Autodesk Inventor part; units mm, degrees
(part 2 of 2)
  line L970 (21.6726, 19.3199) -> (21.796, 19.3518)
  line L971 (21.796, 19.3518) -> (21.9215, 19.3807)
  line L972 (21.9215, 19.3807) -> (22.0489, 19.4065)
  line L973 (22.0489, 19.4065) -> (22.1782, 19.4293)
  line L974 (22.1782, 19.4293) -> (22.4868, 18.9817)
  line L975 (22.4868, 18.9817) -> (22.4196, 18.8689)
  line L976 (22.4196, 18.8689) -> (22.3502, 18.759)
  line L977 (22.3502, 18.759) -> (22.2787, 18.6519)
  line L978 (22.2787, 18.6519) -> (22.2049, 18.5479)
  line L979 (22.2049, 18.5479) -> (22.129, 18.4471)
  line L980 (22.129, 18.4471) -> (22.0506, 18.3498)
  line L981 (22.0506, 18.3498) -> (21.9698, 18.2563)
  line L982 (21.9698, 18.2563) -> (21.8864, 18.1668)
  line L983 (21.8864, 18.1668) -> (21.8436, 18.1237)
  line L984 (21.8436, 18.1237) -> (21.8, 18.0819)
  line L985 (21.8, 18.0819) -> (21.7779, 18.0615)
  line L986 (21.7779, 18.0615) -> (21.7556, 18.0414)
  line L987 (21.7556, 18.0414) -> (21.733, 18.0218)
  line L988 (21.733, 18.0218) -> (21.7101, 18.0026)
  line L989 (21.7101, 18.0026) -> (22.0351, 17.4306)
  line L990 (22.0351, 17.4306) -> (22.0632, 17.4404)
  line L991 (22.0632, 17.4404) -> (22.0917, 17.4497)
  line L992 (22.0917, 17.4497) -> (22.1203, 17.4586)
  line L993 (22.1203, 17.4586) -> (22.1492, 17.4672)
  line L994 (22.1492, 17.4672) -> (22.2074, 17.4832)
  line L995 (22.2074, 17.4832) -> (22.2663, 17.4979)
  line L996 (22.2663, 17.4979) -> (22.3859, 17.5237)
  line L997 (22.3859, 17.5237) -> (22.5077, 17.5452)
  line L998 (22.5077, 17.5452) -> (22.6314, 17.5626)
  line L999 (22.6314, 17.5626) -> (22.7569, 17.5764)
  line L1000 (22.7569, 17.5764) -> (22.884, 17.5865)
  line L1001 (22.884, 17.5865) -> (23.0125, 17.5931)
  line L1002 (23.0125, 17.5931) -> (23.1425, 17.5964)
  line L1003 (23.1425, 17.5964) -> (23.2738, 17.5964)
  line L1004 (23.2738, 17.5964) -> (23.5001, 17.102)
  line L1005 (23.5001, 17.102) -> (23.4143, 17.0026)
  line L1006 (23.4143, 17.0026) -> (23.3269, 16.9063)
  line L1007 (23.3269, 16.9063) -> (23.2379, 16.8134)
  line L1008 (23.2379, 16.8134) -> (23.1472, 16.7238)
  line L1009 (23.1472, 16.7238) -> (23.0548, 16.6378)
  line L1010 (23.0548, 16.6378) -> (22.9608, 16.5555)
  line L1011 (22.9608, 16.5555) -> (22.8649, 16.4774)
  line L1012 (22.8649, 16.4774) -> (22.7672, 16.4037)
  line L1013 (22.7672, 16.4037) -> (22.7176, 16.3687)
  line L1014 (22.7176, 16.3687) -> (22.6674, 16.3351)
  line L1015 (22.6674, 16.3351) -> (22.6421, 16.3188)
  line L1016 (22.6421, 16.3188) -> (22.6166, 16.303)
  line L1017 (22.6166, 16.303) -> (22.591, 16.2876)
  line L1018 (22.591, 16.2876) -> (22.5651, 16.2726)
  line L1019 (22.5651, 16.2726) -> (22.7858, 15.6529)
  line L1020 (22.7858, 15.6529) -> (22.8153, 15.6577)
  line L1021 (22.8153, 15.6577) -> (22.8449, 15.6619)
  line L1022 (22.8449, 15.6619) -> (22.8746, 15.6658)
  line L1023 (22.8746, 15.6658) -> (22.9045, 15.6692)
  line L1024 (22.9045, 15.6692) -> (22.9647, 15.6749)
  line L1025 (22.9647, 15.6749) -> (23.0252, 15.6791)
  line L1026 (23.0252, 15.6791) -> (23.1475, 15.6838)
  line L1027 (23.1475, 15.6838) -> (23.2712, 15.6837)
  line L1028 (23.2712, 15.6837) -> (23.3961, 15.6794)
  line L1029 (23.3961, 15.6794) -> (23.522, 15.6711)
  line L1030 (23.522, 15.6711) -> (23.6489, 15.659)
  line L1031 (23.6489, 15.659) -> (23.7767, 15.6432)
  line L1032 (23.7767, 15.6432) -> (23.9052, 15.6238)
  line L1033 (23.9052, 15.6238) -> (24.0345, 15.601)
  line L1034 (24.0345, 15.601) -> (24.1716, 15.0749)
  line L1035 (24.1716, 15.0749) -> (24.0698, 14.992)
  line L1036 (24.0698, 14.992) -> (23.967, 14.9124)
  line L1037 (23.967, 14.9124) -> (23.8632, 14.8362)
  line L1038 (23.8632, 14.8362) -> (23.7583, 14.7637)
  line L1039 (23.7583, 14.7637) -> (23.6525, 14.695)
  line L1040 (23.6525, 14.695) -> (23.5456, 14.6303)
  line L1041 (23.5456, 14.6303) -> (23.4376, 14.57)
  line L1042 (23.4376, 14.57) -> (23.3286, 14.5144)
  line L1043 (23.3286, 14.5144) -> (23.2737, 14.4886)
  line L1044 (23.2737, 14.4886) -> (23.2184, 14.4642)
  line L1045 (23.2184, 14.4642) -> (23.1907, 14.4526)
  line L1046 (23.1907, 14.4526) -> (23.1628, 14.4414)
  line L1047 (23.1628, 14.4414) -> (23.1349, 14.4307)
  line L1048 (23.1349, 14.4307) -> (23.1068, 14.4204)
  line L1049 (23.1068, 14.4204) -> (23.2165, 13.7718)
  line L1050 (23.2165, 13.7718) -> (23.2464, 13.7714)
  line L1051 (23.2464, 13.7714) -> (23.2763, 13.7705)
  line L1052 (23.2763, 13.7705) -> (23.3063, 13.7691)
  line L1053 (23.3063, 13.7691) -> (23.3363, 13.7672)
  line L1054 (23.3363, 13.7672) -> (23.3965, 13.7624)
  line L1055 (23.3965, 13.7624) -> (23.4569, 13.756)
  line L1056 (23.4569, 13.756) -> (23.5781, 13.7394)
  line L1057 (23.5781, 13.7394) -> (23.6999, 13.7179)
  line L1058 (23.6999, 13.7179) -> (23.8221, 13.692)
  line L1059 (23.8221, 13.692) -> (23.9447, 13.6619)
  line L1060 (23.9447, 13.6619) -> (24.0676, 13.6279)
  line L1061 (24.0676, 13.6279) -> (24.1906, 13.5902)
  line L1062 (24.1906, 13.5902) -> (24.3139, 13.5488)
  line L1063 (24.3139, 13.5488) -> (24.4374, 13.5039)
  line L1064 (24.4374, 13.5039) -> (24.481, 12.9617)
  line L1065 (24.481, 12.9617) -> (24.3665, 12.8976)
  line L1066 (24.3665, 12.8976) -> (24.2514, 12.8371)
  line L1067 (24.2514, 12.8371) -> (24.1359, 12.7801)
  line L1068 (24.1359, 12.7801) -> (24.0201, 12.7269)
  line L1069 (24.0201, 12.7269) -> (23.9039, 12.6777)
  line L1070 (23.9039, 12.6777) -> (23.7874, 12.6325)
  line L1071 (23.7874, 12.6325) -> (23.6706, 12.5919)
  line L1072 (23.6706, 12.5919) -> (23.5536, 12.556)
  line L1073 (23.5536, 12.556) -> (23.495, 12.5401)
  line L1074 (23.495, 12.5401) -> (23.4364, 12.5257)
  line L1075 (23.4364, 12.5257) -> (23.407, 12.5191)
  line L1076 (23.407, 12.5191) -> (23.3776, 12.5129)
  line L1077 (23.3776, 12.5129) -> (23.3483, 12.5072)
  line L1078 (23.3483, 12.5072) -> (23.3189, 12.502)
  line L1079 (23.3189, 12.502) -> (23.3143, 11.8442)
  line L1080 (13.751, 12.2509) -> (13.6999, 12.6391)
  line L1081 (13.6999, 12.6391) -> (13.5499, 13.0009)
  line L1082 (13.5499, 13.0009) -> (13.3115, 13.3115)
  line L1083 (13.3115, 13.3115) -> (13.0009, 13.5499)
  line L1084 (13.0009, 13.5499) -> (12.6391, 13.6998)
  line L1085 (12.6391, 13.6998) -> (12.2509, 13.7509)
  line L1086 (12.2509, 13.7509) -> (11.8626, 13.6998)
  line L1087 (11.8626, 13.6998) -> (11.5009, 13.5499)
  line L1088 (11.5009, 13.5499) -> (11.1902, 13.3115)
  line L1089 (11.1902, 13.3115) -> (10.9518, 13.0009)
  line L1090 (10.9518, 13.0009) -> (10.802, 12.6391)
  line L1091 (10.802, 12.6391) -> (10.7509, 12.2509)
  line L1092 (10.7509, 12.2509) -> (10.802, 11.8626)
  line L1093 (10.802, 11.8626) -> (10.9518, 11.5009)
  line L1094 (10.9518, 11.5009) -> (11.1902, 11.1902)
  line L1095 (11.1902, 11.1902) -> (11.5009, 10.9518)
  line L1096 (11.5009, 10.9518) -> (11.8626, 10.802)
  line L1097 (11.8626, 10.802) -> (12.2509, 10.7509)
  line L1098 (12.2509, 10.7509) -> (12.6391, 10.802)
  line L1099 (12.6391, 10.802) -> (13.0014, 10.952)
  line L1100 (13.0014, 10.952) -> (13.3116, 11.1902)
  line L1101 (13.3116, 11.1902) -> (13.55, 11.5009)
  line L1102 (13.55, 11.5009) -> (13.6998, 11.8626)
  line L1103 (13.6998, 11.8626) -> (13.751, 12.2509)
  point P0 (0, 0)
  constraints: 2208 end point, 438 perpendicular, 117 parallel
extrude "Extrusion1" add sketch "Sketch1" along normal blind 2.5
body "Solid1"
